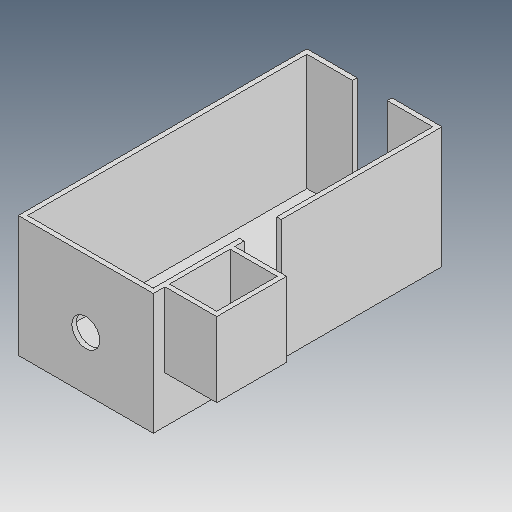
# Autodesk Inventor part: tension_sensor_cover
Saved by Autodesk Inventor 2025.2 (Build 292293000, 293)
## iProperties
Created: 2025-02-17
Part Number: tension_sensor_cover
Material: Generic
Document SubType Name: Modeling
Designer: email
Density: 1 g/cm^3
Appearance: Default
Author: email
Autodesk Inventor part; units mm, degrees
ref_plane "YZ Plane" through (0, 0, 0) normal (1, 0, 0) x (0, 1, 0)
ref_plane "XZ Plane" through (0, 0, 0) normal (0, 1, 0) x (-1, 0, 0)
ref_plane "XY Plane" through (0, 0, 0) normal (0, 0, 1) x (1, 0, 0)
sketch "Sketch1" plane through (0, 0, 0) normal (0, 1, 0) x (-1, 0, 0)
  line L0 (-58, -124) -> (0, -124)
  line L1 (0, -124) -> (0, 0)
  line L2 (-56, -33) -> (-56, -122)
  line L3 (-56, -122) -> (-36.5, -122)
  line L4 (-36.5, -122) -> (-36.5, -124)
  line L5 (-2, -2) -> (-2, -122)
  line L6 (-2, -122) -> (-21.5, -122)
  line L7 (-21.5, -122) -> (-21.5, -124)
  line L8 (-58, -35) -> (-58, -124)
  line L9 (-29, -124) -> (-29, 0) construction
  line L10 (-58, -124) -> (-58, 0)
  line L11 (-56, -124) -> (-56, -2)
  line L12 (-2, -2) -> (-56, -2)
  line L13 (-58, 0) -> (0, 0)
  line L14 (-80.2342, -5) -> (-80.2342, -35)
  line L15 (-80.2342, -35) -> (-56, -35)
  line L16 (-56, -35) -> (-56, 0)
  line L17 (-78.2342, -7) -> (-78.2342, -33)
  line L18 (-78.2342, -33) -> (-56, -33)
  line L19 (-56, -33) -> (-56, -2)
  line L20 (-78.2342, -7) -> (-58, -7)
  line L21 (-80.2342, -5) -> (-58, -5)
  point P0 (-57.4156, -121.9986)
  point P1 (-58, -35)
  point P2 (-58, -38)
  point P3 (-56, -33)
  point P4 (-58, -33)
  dimension "d0" = 58
  dimension "d5" = 2
  dimension "d6" = 15
  dimension "d38" = 2
  dimension "d39" = 58
  dimension "d46" = 2
  dimension "d47" = 2
  dimension "d48" = 2
  dimension "d50" = 30
  dimension "d51" = 2
  constraints: 44 end point, 7 perpendicular, 6 point on line, 3 parallel, 2 collinear, 2 vertical, 1 horizontal, 1 midpoint
  measures "d0" distance of L1.end L10.end
  measures "d5" distance between parallel lines of L0 L6
  measures "d6" distance between parallel lines of L4 L7
  measures "d38" distance between parallel lines of L8 L2
  measures "d39" distance between parallel lines of L1 L8
  measures "d46" distance between parallel lines of L13 L12
  measures "d47" distance between parallel lines of L18 L15
  measures "d48" distance between parallel lines of L14 L17
  measures "d50" distance of L14.start L14.end
  measures "d51" distance between parallel lines of L21 L20
extrude "Extrusion1" add sketch "Sketch1" against normal blind 2 contours L8 L15 L2 L11 L0 | L11 L3 L4 L0 | L10 L18 L2 L15 | L4 L3 L2 L11 L12 L5 L6 L7 L0 | L10 L13 L16 L11 L18 | L7 L6 L5 L12 L16 L13 L1 L0
extrude "Extrusion2" add sketch "Sketch1" along normal blind 50 contours L8 L15 L2 L11 L0 | L11 L3 L4 L0 | L10 L18 L2 L15 | L10 L13 L16 L11 L18 | L7 L6 L5 L12 L16 L13 L1 L0
sketch "Sketch2" plane through (0, -2, 0) normal (0, 0, 1) x (1, 0, 0)
  circle A0 centre (29, 23) radius 6
  line L0 (-8.0985, 48) -> (58, 48) projected
  line L1 (58, 0) -> (58, 52) projected
  point P0 (0, 2)
  point P1 (0, 52)
  point P2 (29, 48)
  point P3 (66.0985, 48)
  dimension "d11" = 25
  dimension "d12" = 12
  constraints: 1 centre point, 1 vertical alignment, 2 other
  measures "d12" diameter of A0
extrude "Extrusion3" cut sketch "Sketch2" against normal up to next
sketch "Sketch3" plane through (58, -2, 5.4121) normal (1, 0, 0) x (0, 0, -1)
  arc A0 (44.4121, 16) -> (60.4121, 16) centre (52.4121, 16) ccw
  line L0 (5.4121, 1.9762) -> (5.4121, 47)
  line L1 (60.4121, 16) -> (60.4121, 61)
  line L2 (60.4121, 61) -> (44.4121, 61)
  line L3 (44.4121, 61) -> (44.4121, 16)
  line L4 (5.4121, 47) -> (129.4107, 47) construction
  point P0 (5.4121, 2)
  point P1 (129.4107, 47)
  point P2 (5.4121, 0)
  dimension "d16" = 47
  dimension "d17" = 16
  dimension "d18" = 31
  dimension "d45" = 45
  constraints: 8 end point, 2 point on circle, 2 tangent, 2 vertical, 1 centre point, 1 parallel, 1 perpendicular, 1 point on line, 3 other
  measures "d16" distance from line of L0 A0.centre
  measures "d17" diameter of A0
  measures "d45" distance of L1.start L1.end
extrude "Extrusion4" cut sketch "Sketch3" against normal blind 2
ref_plane "Work Plane1" through (0, 18, 0) normal (0, -1, 0) x (1, 0, 0)
extrude "Extrusion7" add sketch "Sketch1" along normal up to surface (32 mm away) from surface at 18 contours L15 L14 L21 L10 L20 L17 L18
body "Solid1"
